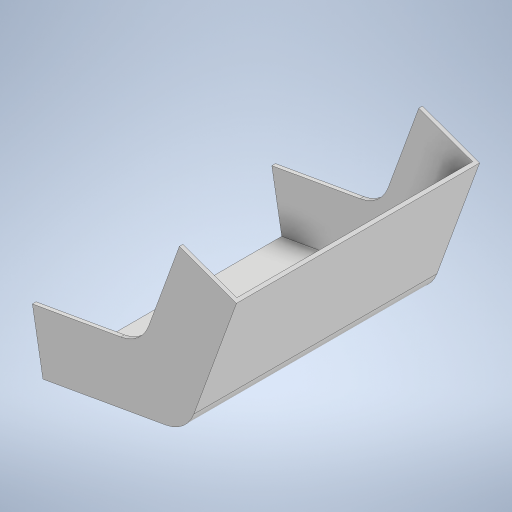
# Autodesk Inventor part: splitter
Saved by Autodesk Inventor 2023 (Build 270158000, 158)
## iProperties
Created: 2023-06-06
Part Number: splitter
Material: 一般
Document SubType Name: Modeling
Designer: USER
Density: 1 g/cm^3
Appearance: 預設
Author: USER
Autodesk Inventor part; units mm, degrees
ref_plane "YZ Plane" through (0, 0, 0) normal (1, 0, 0) x (0, 1, 0)
ref_plane "XZ Plane" through (0, 0, 0) normal (0, 1, 0) x (-1, 0, 0)
ref_plane "XY Plane" through (0, 0, 0) normal (0, 0, 1) x (1, 0, 0)
sketch "草圖1" plane through (0, 0, 0) normal (0, 0, 1) x (1, 0, 0)
  line L0 (0, 0) -> (-118.1769, -20.8378)
  line L1 (0, 0) -> (41.0424, 112.7631)
  line L2 (-150.6339, 0) -> (72.9885, 0) projected
  line L3 (-1.9284, 2.2981) -> (38.2199, 113.7796)
  line L4 (-1.9284, 2.2981) -> (-118.6879, -17.8816)
  line L5 (0, 0) -> (-1.9284, 2.2981) construction
  line L6 (-118.6879, -17.8816) -> (-118.1769, -20.8378)
  line L7 (38.2199, 113.7796) -> (41.0424, 112.7631)
  dimension "d0" = 10
  dimension "d1" = 70
  dimension "d2" = 120
  dimension "d3" = 60
  dimension "d5" = 3
  constraints: 14 end point, 3 equal length, 2 perpendicular
  measures "d0" angle of L2 L0
  measures "d1" angle of L2 L1
  measures "d2" distance of L0.start L1.end
  measures "d3" angle of L1 L5
  measures "d5" distance of L3.end L1.end
extrude "擠出1" add sketch "草圖1" along normal blind 200
sketch "草圖2" plane through (0, 0, 200) normal (0, 0, 1) x (1, 0, 0)
  line L0 (-118.1769, -20.8378) -> (0, 0) projected
  line L1 (0, 0) -> (41.0424, 112.7631) projected
  line L2 (41.0424, 112.7631) -> (38.2199, 113.7796) projected
  line L3 (38.2199, 113.7796) -> (-1.9284, 2.2981) projected
  line L4 (-1.9284, 2.2981) -> (-118.6879, -17.8816) projected
  line L5 (-118.6879, -17.8816) -> (-118.1769, -20.8378) projected
  line L6 (-118.1769, -20.8378) -> (0, 0)
  line L7 (0, 0) -> (41.0424, 112.7631)
  line L8 (-126.8593, 28.4026) -> (-37.1114, 44.2276)
  line L9 (-37.1114, 44.2276) -> (-5.9422, 129.8641)
  line L10 (-37.1114, 44.2276) -> (0, 0) construction
  line L11 (-126.8593, 28.4026) -> (-118.1769, -20.8378)
  line L12 (-5.9422, 129.8641) -> (41.0424, 112.7631)
  dimension "d9" = 60
  dimension "d10" = 50
  constraints: 14 end point, 3 parallel, 2 perpendicular, 1 collinear
  measures "d9" angle of L1 L10
  measures "d10" distance of L9.end L1.end
extrude "擠出2" add sketch "草圖2" against normal blind 200 contours L11 L8 L9 L12 L2 L3 L4 L5
shell "薄殼1" thickness 3 removed faces 4 at (-16.3319, 101.3186, 133.3333) at (25.3809, 118.4635, 133.3333) at (-67.0274, 38.9526, 133.3333) at (-123.9652, 11.9891, 133.3333)
fillet "圓角2" radius 30 4 edges at (-2.2267, 2.6537, 100) (0, 0, 100) (-37.1114, 44.2276, 198.5) (-37.1114, 44.2276, 1.5)
